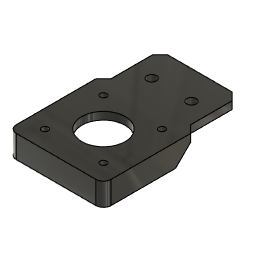
3030 AB Motor Bracket_2x (Autodesk Fusion 360 design; units mm, degrees)
Autodesk Fusion 360 part; units mm, degrees
sketch "Sketch1" plane through (0, 0, 0) normal (0, 0, 1) x (1, 0, 0)
  circle A0 centre (0, 0) radius 6.11 construction
  line L0 (15.5, -15.5) -> (-15.5, -15.5) construction
  line L1 (-15.5, -15.5) -> (-15.5, 15.5) construction
  line L2 (-15.5, 15.5) -> (15.5, 15.5) construction
  line L3 (15.5, 15.5) -> (15.5, -15.5) construction
  line L4 (15.5, -15.5) -> (-15.5, 15.5) construction
  line L5 (-15.5, -15.5) -> (15.5, 15.5) construction
  circle A1 centre (0, 0) radius 11.5
  line L6 (-21.1, 21.1) -> (21.1, 21.1) construction
  line L7 (21.1, 21.1) -> (21.1, -21.1)
  line L8 (21.1, -21.1) -> (-21.1, -21.1)
  line L9 (-21.1, -21.1) -> (-21.1, 21.1)
  line L10 (0, 21.1) -> (0, -21.1) construction
  line L11 (-21.1, 21.1) -> (21.1, 21.1) construction
  line L12 (21.1, 21.1) -> (21.1, 51.1)
  line L13 (21.1, 51.1) -> (-21.1, 51.1)
  line L14 (-21.1, 51.1) -> (-21.1, 21.1)
  line L15 (0, 51.1) -> (0, 36.1) construction
  line L16 (0, 36.1) -> (21.1, 36.1) construction
  circle A2 centre (10.55, 36.1) radius 2.5
  circle A3 centre (-10.55, 36.1) radius 2.5
  line L17 (-25.1, 25.1) -> (25.1, 25.1) construction
  line L18 (25.1, 25.1) -> (25.1, -25.1)
  line L19 (25.1, -25.1) -> (-25.1, -25.1)
  line L20 (-25.1, -25.1) -> (-25.1, 25.1)
  line L21 (-25.1, 21.1) -> (25.1, 21.1)
  dimension "d5021" = 12.22
  dimension "d5033" = 31
  dimension "d5091" = 23
  dimension "d5656" = 42.2
  dimension "d5657" = 42.2
  dimension "d5659" = 30
  dimension "d5660" = 5
  constraint horizontal L0
  constraint perpendicular L0 L1
  constraint parallel L0 L2
  constraint parallel L1 L3
  constraint coincident L4 A0.centre
  constraint coincident L5 A0.centre
  constraint coincident A0.centre A1.centre
  constraint concentric A0 A1
  constraint equal L0 L1
  constraint horizontal L6
  constraint vertical L7
  constraint horizontal L8
  constraint vertical L9
  constraint midpoint L6 L10.start
  constraint midpoint L8 L10.end
  constraint midpoint A0.centre L10
  constraint horizontal L11
  constraint vertical L12
  constraint horizontal L13
  constraint vertical L14
  constraint coincident L6.end L7.start
  constraint midpoint L13 L15.start
  constraint perpendicular L13 L15
  constraint perpendicular L12 L16
  constraint midpoint L12 L16.end
  constraint midpoint L16 A2.centre
  constraint symmetric L15 A2 A3
  constraint coincident L20 L21.start
  constraint coincident L18 L21.end
  constraint perpendicular L18 L21
  constraint coincident L10.start L21
  measures "d5021" diameter of A0
  measures "d5033" distance of L0.end L1.end
  measures "d5091" diameter of A1
  measures "d5656" distance of L6.start L6.end
  measures "d5657" distance of L6.start L8.end
  measures "d5659" distance of L6.start L13.end
  measures "d5660" diameter of A2
extrude "Extrude1" add sketch "Sketch1" along normal blind 4 contours L12 L13 L14 L21 | L7 L8 L9 L21
extrude "Extrude12" add sketch "Sketch1" along normal up to surface (4 mm away) and the other way blind 8 contours L7 L8 L9 L18 L19 L20 L21
hole "Hole1" at (15.5, 15.5, 0) at (15.5, -15.5, 0) at (-15.5, -15.5, 0) at (-15.5, 15.5, 0) direction (0, 0, 1) diameter 3.4 depth 35 tip angle 118
chamfer "Chamfer5" distance 4 angle 45 4 edges at (21.1, 51.1, 2) (-21.1, 51.1, 2) (21.1, 21.1, 2) (-21.1, 21.1, 2)
chamfer "Chamfer5" distance 8 angle 45 2 edges at (23.1, 21.1, -8) (-23.1, 21.1, -8)
fillet "Fillet2" radius 4 2 edges at (25.1, -25.1, -2) (-25.1, -25.1, -2)
equation "d4171 = Part_Thickness"
equation "d5021 = Pulley_od"
equation "d5656 = d5657"
equation "d5661 = -Part_Thickness"
equation "Part_Thickness = 4 mm" comment "Thickness of Printed Parts"
equation "Pulley_od = 12.22 mm" comment "GT2 Pulley/Idler Tooth OD"
